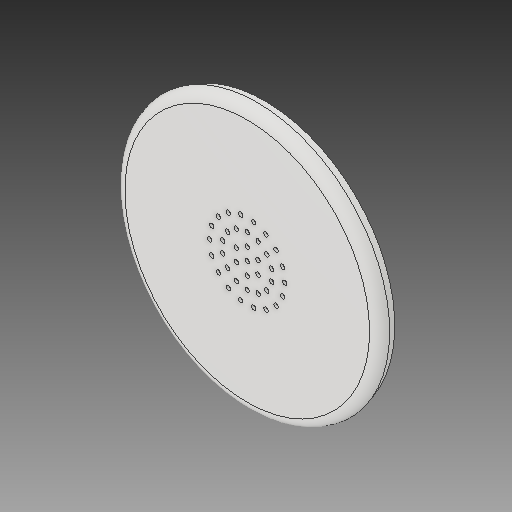
# Autodesk Inventor part: lid_top
Saved by Autodesk Inventor 2017 (Build 210142000, 142)
## iProperties
Created: 2016-09-25
Part Number: lid_top
Material: PC/ABS Plastic
Document SubType Name: Modeling
Designer: Jason
Density: 0.357273 g/cm^3
Appearance: Smooth - White
Author: Jason
Autodesk Inventor part; units mm, degrees
ref_plane "YZ Plane" through (0, 0, 0) normal (1, 0, 0) x (0, 1, 0)
ref_plane "XZ Plane" through (0, 0, 0) normal (0, 1, 0) x (-1, 0, 0)
ref_plane "XY Plane" through (0, 0, 0) normal (0, 0, 1) x (1, 0, 0)
sketch "Sketch1" plane through (0, 0, 0) normal (0, 0, 1) x (1, 0, 0)
  circle A0 centre (0, 0) radius 52.75
  dimension "d0" = 105.5
  constraints: 1 centre point, 1 coincident
  measures "d0" diameter of A0
extrude "Extrusion1" add sketch "Sketch1" along normal blind 7
fillet "Fillet1" radius 4 1 edges at (-52.75, 0, 7)
sketch "Sketch2" plane through (0, 0, 0) normal (0, 0, -1) x (-1, 0, 0)
  circle A0 centre (0, 0) radius 51.8
  circle A1 centre (0, 0) radius 52.75
  circle A2 centre (0, 0) radius 52.75 projected
  dimension "d4" = 103.6
  dimension "d69" = 0
  constraints: 2 centre point, 2 coincident
  measures "d4" diameter of A0
  measures "d69" radial gap between concentric circles of A2 A1
extrude "Extrusion2" cut sketch "Sketch2" against normal blind 3
sketch "Sketch3" plane through (0, 0, 0) normal (0, 0, -1) x (-1, 0, 0)
  circle A0 centre (0, 0) radius 48.75
  constraints: 1 centre point, 1 coincident
extrude "Extrusion3" cut sketch "Sketch3" against normal blind 6
sketch "Sketch6" plane through (0, 0, 7) normal (0, 0, 1) x (1, 0, 0)
  circle A0 centre (0, 0) radius 15 construction
  circle A1 centre (15, 0) radius 1
  circle A2 centre (14.0954, 5.1303) radius 1
  circle A3 centre (11.4907, 9.6418) radius 1
  circle A4 centre (7.5, 12.9904) radius 1
  circle A5 centre (2.6047, 14.7721) radius 1
  circle A6 centre (-2.6047, 14.7721) radius 1
  circle A7 centre (-7.5, 12.9904) radius 1
  circle A8 centre (-11.4907, 9.6418) radius 1
  circle A9 centre (-14.0954, 5.1303) radius 1
  circle A10 centre (-15, 0) radius 1
  circle A11 centre (-14.0954, -5.1303) radius 1
  circle A12 centre (-11.4907, -9.6418) radius 1
  circle A13 centre (-7.5, -12.9904) radius 1
  circle A14 centre (-2.6047, -14.7721) radius 1
  circle A15 centre (2.6047, -14.7721) radius 1
  circle A16 centre (7.5, -12.9904) radius 1
  circle A17 centre (11.4907, -9.6418) radius 1
  circle A18 centre (14.0954, -5.1303) radius 1
  circle A19 centre (0, 0) radius 10 construction
  circle A20 centre (0, -10) radius 1
  circle A21 centre (4.3388, -9.0097) radius 1
  circle A22 centre (7.8183, -6.2349) radius 1
  circle A23 centre (9.7493, -2.2252) radius 1
  circle A24 centre (9.7493, 2.2252) radius 1
  circle A25 centre (7.8183, 6.2349) radius 1
  circle A26 centre (4.3388, 9.0097) radius 1
  circle A27 centre (0, 10) radius 1
  circle A28 centre (-4.3388, 9.0097) radius 1
  circle A29 centre (-7.8183, 6.2349) radius 1
  circle A30 centre (-9.7493, 2.2252) radius 1
  circle A31 centre (-9.7493, -2.2252) radius 1
  circle A32 centre (-7.8183, -6.2349) radius 1
  circle A33 centre (-4.3388, -9.0097) radius 1
  circle A34 centre (0, 0) radius 5 construction
  circle A35 centre (0, -5) radius 1
  circle A36 centre (4.3301, -2.5) radius 1
  circle A37 centre (4.3301, 2.5) radius 1
  circle A38 centre (0, 5) radius 1
  circle A39 centre (-4.3301, 2.5) radius 1
  circle A40 centre (-4.3301, -2.5) radius 1
  dimension "d44" = 30
  dimension "d50" = 20
  dimension "d56" = 10
  dimension "d45" = 2
  dimension "d48" = 360
  dimension "d51" = 2
  dimension "d54" = 360
  dimension "d57" = 2
  dimension "d60" = 360
  constraints: 38 centre point, 3 coincident, 2 vertical alignment, 1 horizontal alignment, 85 other
  measures "d45" diameter of A1
  measures "d51" diameter of A20
  measures "d57" diameter of A35
hole "Hole1" at (0, 5, 7) at (0, 10, 7) at (4.3388, 9.0097, 7) at (7.8183, 6.2349, 7) at (7.5, 12.9904, 7) at (4.3301, 2.5, 7) at (9.7493, 2.2252, 7) at (0, 0, 7) at (0, 0, 7) at (0, 0, 7) at (4.3301, -2.5, 7) at (-7.8183, 6.2349, 7) at (-4.3301, -2.5, 7) at (0, -5, 7) at (0, 0, 7) at (15, 0, 7) at (14.0954, 5.1303, 7) at (11.4907, 9.6418, 7) at (2.6047, 14.7721, 7) at (-4.3388, 9.0097, 7) at (-11.4907, 9.6418, 7) at (-7.5, 12.9904, 7) at (-2.6047, 14.7721, 7) at (11.4907, -9.6418, 7) at (9.7493, -2.2252, 7) at (7.8183, -6.2349, 7) at (14.0954, -5.1303, 7) at (-14.0954, 5.1303, 7) at (-15, 0, 7) at (-14.0954, -5.1303, 7) at (-11.4907, -9.6418, 7) at (-7.5, -12.9904, 7) at (-4.3301, 2.5, 7) at (-4.3388, -9.0097, 7) at (-7.8183, -6.2349, 7) at (-9.7493, 2.2252, 7) at (-9.7493, -2.2252, 7) at (-2.6047, -14.7721, 7) at (2.6047, -14.7721, 7) at (7.5, -12.9904, 7) at (4.3388, -9.0097, 7) at (0, -10, 7) direction (0, 0, -1) diameter 1.778 depth 10.688
fillet "Fillet2" radius 2 1 edges at (48.75, 0, 6)
body "Solid1"
